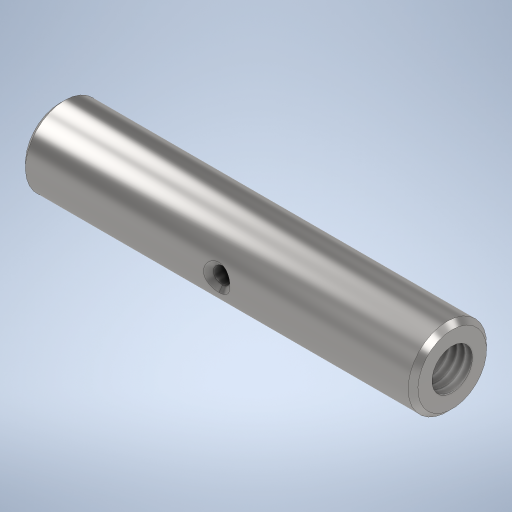
# Autodesk Inventor part: bolt_V1
Saved by Autodesk Inventor 2023 (Build 270158000, 158)
## iProperties
Created: 2023-05-10
Part Number: bolt_V1
Material: Stahl, Legierung
Document SubType Name: Modeling
Designer: Mathi
Density: 7.73 g/cm^3
Appearance: Halbpoliert
Author: Mathi
Autodesk Inventor part; units mm, degrees
ref_plane "YZ Plane" through (0, 0, 0) normal (1, 0, 0) x (0, 1, 0)
ref_plane "XZ Plane" through (0, 0, 0) normal (0, 1, 0) x (-1, 0, 0)
ref_plane "XY Plane" through (0, 0, 0) normal (0, 0, 1) x (1, 0, 0)
sketch "Skizze1" plane through (0, 0, 0) normal (0, 0, 1) x (1, 0, 0)
  line L0 (0, 0) -> (24.9383, 0)
  line L1 (20, 0) -> (-20, 0)
  line L2 (-20, 0) -> (-20, 4)
  line L3 (-20, 4) -> (20, 4)
  line L4 (20, 4) -> (20, 0)
  circle A0 centre (0, 0) radius 0.85
  dimension "d0" = 40
  dimension "d1" = 8
  dimension "d2" = 1.7
  constraints: 10 end point, 2 horizontal, 2 parallel, 1 centre point, 1 coincident, 1 midpoint, 1 perpendicular, 1 point on line
  measures "d0" distance of L2.end L3.end
  measures "d1" diameter of L3 L0
  measures "d2" diameter of A0
revolve "Umdrehung1" add sketch "Skizze1" angle 360 about axis through (0, 0, 0) along (1, 0, 0) picked at (-0.5584, 0.0678) contours L1 A0 L0 | A0 L1 L2 L3 L4 L0
sketch "Skizze2" plane through (0, 0, 0) normal (0, 0, 1) x (1, 0, 0)
  circle A0 centre (0, 0) radius 0.85 projected
extrude "Extrusion1" cut sketch "Skizze2" along normal through all both and the other way through all
sketch "Skizze3" plane through (20, 0, 0) normal (1, 0, 0) x (0, 0, -1)
  point P0 (0, 0)
  point P1 (0, 0)
  constraints: 1 coincident
hole "Bohrung1" at (20, 0, 0) direction (-1, 0, 0) diameter 4.134 depth 21 tip angle 118 thread size "M5x0.8" class "6H" standard "ISO Metric profile"
chamfer "Fase1" distance 0.5 angle 45 2 edges at (20, -4, 0) (-20, -4, 0)
chamfer "Fase2" distance 0.5 angle 45 2 edges at (-0.85, -0.0027, 4) (-0.85, -0.0027, -4)
